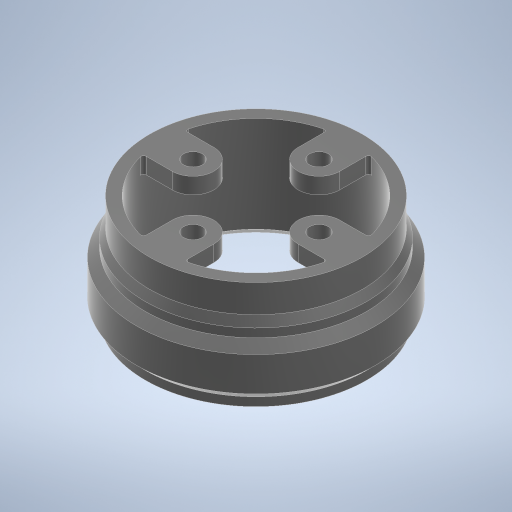
# Autodesk Inventor part: Motor Hub
Saved by Autodesk Inventor 2023.2 (Build 272271000, 271)
## iProperties
Created: 2022-12-29
Part Number: Motor Hub
Material: Nylon 6/6
Document SubType Name: Modeling
Designer: Nathan Cai
Density: 1.13 g/cm^3
Appearance: Smooth - Black
Mass: 9.71742 g
Surface Area: 89.0077 cm^2
Volume: 8.59949 cm^3
Author: Nathan Cai
Autodesk Inventor part; units mm, degrees
ref_plane "YZ Plane" through (0, 0, 0) normal (1, 0, 0) x (0, 1, 0)
ref_plane "XZ Plane" through (0, 0, 0) normal (0, 1, 0) x (-1, 0, 0)
sketch "Sketch1" plane through (0, 0, 0) normal (0, 1, 0) x (-1, 0, 0)
  circle A0 centre (0, 0) radius 22.225 construction
  circle A1 centre (0, 0) radius 17.65
  circle A2 centre (0, 0) radius 22.225
  dimension "d0" = 44.45
  dimension "d1" = 35.3
  dimension "d2" = 44.45
  constraints: 3 centre point, 3 coincident
  measures "d0" diameter of A0
  measures "d1" diameter of A1
  measures "d2" diameter of A2
extrude "Extrusion1" add sketch "Sketch1" along normal blind 9.525
sketch "Sketch2" plane through (0, 0, 0) normal (0, -1, 0) x (1, 0, 0)
  circle A0 centre (0, 0) radius 17.6
  circle A1 centre (0, 0) radius 20.6375
  dimension "d5" = 41.275
  dimension "d6" = 35.2
  constraints: 2 centre point, 2 coincident
  measures "d5" diameter of A1
  measures "d6" diameter of A0
extrude "Extrusion2" add sketch "Sketch2" along normal blind 1.5875
sketch "Sketch3" plane through (0, 9.525, 0) normal (0, 1, 0) x (1, 0, 0)
  circle A0 centre (0, 0) radius 17.65
  circle A1 centre (0, 0) radius 20.6375
  dimension "d9" = 35.3
  dimension "d10" = 41.275
  constraints: 2 centre point, 2 coincident
  measures "d9" diameter of A0
  measures "d10" diameter of A1
extrude "Extrusion3" add sketch "Sketch3" along normal blind 1.5875
sketch "Sketch4" plane through (0, 0, 0) normal (1, 0, 0) x (0, 1, 0)
  line L0 (11.1125, -17.65) -> (17.8875, -17.65)
  line L1 (17.8875, -17.65) -> (17.8875, -20.6375)
  line L2 (17.8875, -20.6375) -> (11.1125, -20.6375) construction
  line L3 (11.1125, -20.6375) -> (11.1125, -17.65)
  line L4 (11.1125, -20.6375) -> (11.1125, 20.6375) projected
  line L5 (12.7, -17.65) -> (12.7, -20.6375) construction
  line L6 (11.1125, -20.6375) -> (12.7, -19.8438)
  line L7 (12.7, -19.8438) -> (17.8875, -19.8438)
  line L8 (0, 0) -> (25.7056, 0) construction
  line L9 (-11.1125, 0) -> (-11.1125, -19.8438) construction
  line L10 (0, 20.6375) -> (0, -20.6375) projected
  dimension "d13" = 17.65
  dimension "d14" = 20.6375
  dimension "d16" = 1.5875
  dimension "d18" = 19.8438
  dimension "d84" = 11.1125
  dimension "d85" = 29
  constraints: 18 end point, 5 point on line, 3 parallel, 2 horizontal, 2 perpendicular, 1 vertical
  measures "d13" distance from line of L8.start L0
  measures "d14" distance from line of L8.start L2
  measures "d16" distance between parallel lines of L3 L5
  measures "d18" vertical distance of L8.start L7.end
  measures "d84" distance between parallel lines of L9 L10
  measures "d85" distance between parallel lines of L9 L1
revolve "Revolution1" add sketch "Sketch4" angle 360 about axis through (0, 0, 0) along (0, 1, 0)
ref_plane "Work Plane1" through (0, 4.7625, 0) normal (0, 1, 0) x (1, 0, 0)
sketch "Sketch11" plane through (0, 17.8875, 0) normal (0, 1, 0) x (1, 0, 0)
  circle A0 centre (0, 0) radius 11.75 construction
  line L0 (0, 0) -> (-11.75, 0) construction
  circle A1 centre (-11.75, 0) radius 3.875
  line L1 (-11.75, -3.875) -> (-18.1, -3.875)
  line L2 (-18.1, -3.875) -> (-18.1, 3.875)
  line L3 (-18.1, 3.875) -> (-11.75, 3.875)
  line L4 (-11.75, 3.875) -> (-11.75, -3.875) construction
  circle A2 centre (0, -11.75) radius 3.875
  line L5 (3.875, -11.75) -> (3.875, -18.1)
  line L6 (3.875, -18.1) -> (-3.875, -18.1)
  line L7 (-3.875, -18.1) -> (-3.875, -11.75)
  line L8 (-3.875, -11.75) -> (3.875, -11.75) construction
  circle A3 centre (11.75, 0) radius 3.875
  line L9 (11.75, 3.875) -> (18.1, 3.875)
  line L10 (18.1, 3.875) -> (18.1, -3.875)
  line L11 (18.1, -3.875) -> (11.75, -3.875)
  line L12 (11.75, -3.875) -> (11.75, 3.875) construction
  circle A4 centre (0, 11.75) radius 3.875
  line L13 (-3.875, 11.75) -> (-3.875, 18.1)
  line L14 (-3.875, 18.1) -> (3.875, 18.1)
  line L15 (3.875, 18.1) -> (3.875, 11.75)
  line L16 (3.875, 11.75) -> (-3.875, 11.75) construction
  circle A5 centre (0, -11.75) radius 1.7526
  circle A6 centre (11.75, 0) radius 1.7526
  circle A7 centre (0, 11.75) radius 1.7526
  circle A8 centre (-11.75, 0) radius 1.7526
  point P0 (3.875, 11.75)
  point P1 (11.75, -3.875)
  point P2 (-3.875, -11.75)
  point P3 (-11.75, 3.875)
  dimension "d121" = 23.5
  dimension "d122" = 7.75
  dimension "d123" = 6.35
  dimension "d126" = 360
  dimension "d134" = 3.5052
  dimension "d137" = 360
  constraints: 34 end point, 6 coincident, 4 centre point, 4 horizontal, 2 parallel, 1 horizontal alignment, 1 perpendicular, 68 other
  measures "d123" distance of L2.end L3.end
  measures "d134" diameter of A5
extrude "Extrusion10" add sketch "Sketch11" against normal blind 3
fillet "Fillet5" radius 0.5 8 edges at (-17.2194, 16.3875, -3.875) (-17.2194, 16.3875, 3.875) (-3.875, 16.3875, 17.2194) (3.875, 16.3875, 17.2194) (17.2194, 16.3875, -3.875) (17.2194, 16.3875, 3.875) (-3.875, 16.3875, -17.2194) (3.875, 16.3875, -17.2194)
chamfer "Chamfer5" distance 1.5875 angle 45 1 edges at (-17.6, -1.5875, 0)
chamfer "Chamfer6" distance 1.5875 angle 45 2 edges at (22.225, 9.525, 0) (22.225, 0, 0)
body "Solid1"
